Autodesk Fusion 360 part; units mm, degrees
note: some values were not read from the file. Chosen so that the rebuilt part matches the saved one: which bodies a step acts on; which pieces of a blend or face edit are solid. Set by a fixed rule: which sketch regions a step uses.
(part 4 of 4)
  spline S28 degree 5 poles (-8.8975, 18.3699) (-8.9029, 18.3732) (-8.9137, 18.3794) (-8.9303, 18.3884) (-8.9529, 18.3994) (-8.9818, 18.4118) (-9.0111, 18.4234) (-9.0408, 18.4344) (-9.0706, 18.4451) (-9.1006, 18.4555) (-9.1307, 18.4658) (-9.1609, 18.4758) (-9.1914, 18.4854) (-9.222, 18.4945) (-9.2529, 18.5032) (-9.284, 18.5115) (-9.3152, 18.5194) (-9.3466, 18.527) (-9.3782, 18.5343) (-9.4098, 18.5413) (-9.4416, 18.5482) (-9.4735, 18.5547) (-9.5055, 18.5609) (-9.5376, 18.5669) (-9.5699, 18.5726) (-9.6023, 18.578) (-9.6348, 18.5831) (-9.6674, 18.588) (-9.7002, 18.5926) (-9.733, 18.597) (-9.7659, 18.6011) (-9.7989, 18.605) (-9.832, 18.6087) (-9.8652, 18.6121) (-9.8985, 18.6152) (-9.9319, 18.6182) (-9.9654, 18.6209) (-9.9989, 18.6233) (-10.0326, 18.6256) (-10.0663, 18.6276) (-10.1001, 18.6294) (-10.134, 18.631) (-10.1679, 18.6323) (-10.2019, 18.6334) (-10.236, 18.6344) (-10.2702, 18.635) (-10.3044, 18.6355) (-10.3387, 18.6358) (-10.3731, 18.6358) (-10.4075, 18.6357) (-10.442, 18.6353) (-10.4766, 18.6347) (-10.5112, 18.6339) (-10.5459, 18.6329) (-10.5806, 18.6317) (-10.6154, 18.6303) (-10.6503, 18.6287) (-10.6852, 18.6269) (-10.7202, 18.6249) (-10.7552, 18.6227) (-10.7902, 18.6203) (-10.8253, 18.6176) (-10.8605, 18.6148) (-10.8957, 18.6118) (-10.931, 18.6086) (-10.9663, 18.6052) (-11.0016, 18.6016) (-11.037, 18.5978) (-11.0724, 18.5938) (-11.1079, 18.5896) (-11.1434, 18.5852) (-11.1718, 18.5816) (-11.1932, 18.5787) (-11.2074, 18.5768) (-11.2145, 18.5758) knots 0 0 0 0 0 0 0.01428571 0.02857143 0.04285714 0.05714286 0.07142857 0.08571429 0.1 0.11428571 0.12857143 0.14285714 0.15714286 0.17142857 0.18571429 0.2 0.21428571 0.22857143 0.24285714 0.25714286 0.27142857 0.28571429 0.3 0.31428571 0.32857143 0.34285714 0.35714286 0.37142857 0.38571429 0.4 0.41428571 0.42857143 0.44285714 0.45714286 0.47142857 0.48571429 0.5 0.51428571 0.52857143 0.54285714 0.55714286 0.57142857 0.58571429 0.6 0.61428571 0.62857143 0.64285714 0.65714286 0.67142857 0.68571429 0.7 0.71428571 0.72857143 0.74285714 0.75714286 0.77142857 0.78571429 0.8 0.81428571 0.82857143 0.84285714 0.85714286 0.87142857 0.88571429 0.9 0.91428571 0.92857143 0.94285714 0.95714286 0.97142857 0.98571429 1 1 1 1 1 1
  arc A58 (-11.2145, 18.5758) -> (-11.6071, 17.6942) centre (0, 13.0546) ccw
  spline S29 degree 5 poles (-11.6071, 17.6942) (-11.603, 17.6883) (-11.5949, 17.6764) (-11.5827, 17.6586) (-11.5664, 17.6351) (-11.5459, 17.6057) (-11.5253, 17.5766) (-11.5046, 17.5476) (-11.4837, 17.5187) (-11.4628, 17.4901) (-11.4417, 17.4616) (-11.4205, 17.4332) (-11.3991, 17.405) (-11.3777, 17.377) (-11.3562, 17.3492) (-11.3345, 17.3215) (-11.3127, 17.294) (-11.2908, 17.2667) (-11.2688, 17.2395) (-11.2467, 17.2125) (-11.2244, 17.1857) (-11.2021, 17.1591) (-11.1796, 17.1327) (-11.157, 17.1064) (-11.1344, 17.0803) (-11.1115, 17.0545) (-11.0886, 17.0288) (-11.0656, 17.0032) (-11.0424, 16.9779) (-11.0192, 16.9528) (-10.9958, 16.9279) (-10.9723, 16.9031) (-10.9487, 16.8786) (-10.925, 16.8543) (-10.9011, 16.8302) (-10.8772, 16.8063) (-10.8531, 16.7825) (-10.829, 16.759) (-10.8047, 16.7358) (-10.7803, 16.7127) (-10.7558, 16.6898) (-10.7311, 16.6672) (-10.7064, 16.6448) (-10.6815, 16.6227) (-10.6565, 16.6007) (-10.6314, 16.5791) (-10.6062, 16.5576) (-10.5809, 16.5364) (-10.5554, 16.5154) (-10.5299, 16.4947) (-10.5042, 16.4742) (-10.4784, 16.454) (-10.4524, 16.4341) (-10.4264, 16.4145) (-10.4002, 16.3952) (-10.3738, 16.3761) (-10.3474, 16.3573) (-10.3209, 16.3388) (-10.2942, 16.3205) (-10.2674, 16.3026) (-10.2405, 16.285) (-10.2134, 16.2679) (-10.1861, 16.2512) (-10.1586, 16.235) (-10.1309, 16.2192) (-10.1032, 16.2037) (-10.0753, 16.1885) (-10.0474, 16.1735) (-10.0194, 16.1588) (-9.9912, 16.1447) (-9.9626, 16.1316) (-9.9393, 16.1221) (-9.9216, 16.1158) (-9.9096, 16.1119) (-9.9036, 16.1101) knots -1 -1 -1 -1 -1 -1 -0.98571429 -0.97142857 -0.95714286 -0.94285714 -0.92857143 -0.91428571 -0.9 -0.88571429 -0.87142857 -0.85714286 -0.84285714 -0.82857143 -0.81428571 -0.8 -0.78571429 -0.77142857 -0.75714286 -0.74285714 -0.72857143 -0.71428571 -0.7 -0.68571429 -0.67142857 -0.65714286 -0.64285714 -0.62857143 -0.61428571 -0.6 -0.58571429 -0.57142857 -0.55714286 -0.54285714 -0.52857143 -0.51428571 -0.5 -0.48571429 -0.47142857 -0.45714286 -0.44285714 -0.42857143 -0.41428571 -0.4 -0.38571429 -0.37142857 -0.35714286 -0.34285714 -0.32857143 -0.31428571 -0.3 -0.28571429 -0.27142857 -0.25714286 -0.24285714 -0.22857143 -0.21428571 -0.2 -0.18571429 -0.17142857 -0.15714286 -0.14285714 -0.12857143 -0.11428571 -0.1 -0.08571429 -0.07142857 -0.05714286 -0.04285714 -0.02857143 -0.01428571 0 0 0 0 0 0
  line L29 (-9.9036, 16.1101) -> (-9.6476, 16.0311)
  arc A59 (-9.1027, 15.0919) -> (-9.6476, 16.0311) centre (-9.8834, 15.2666) ccw
  circle A60 centre (0, 13.0546) radius 2
  line L30 (-1.664, 11.945) -> (1.836, 11.945)
  dimension "d55" = 4
  dimension "d56" = 3.5
  constraint concentric A0 A60
  constraint coincident A60 L30.start
  constraint horizontal L30
  measures "d55" diameter of A60
  measures "d56" distance of L30.start L30.end
extrude "Extrude13" cut sketch "Sketch8" against normal blind 4 contours A60 L30 picked at (0.1008, 13.0647) bodies 2
move_body "Move12" bodies 2 to x (1, 0, 0) y (0, 0, -1) z (0, 1, 0) at (0, 0, 0)
move_body "Move13" bodies 2 to x (1, 0, 0) y (0, 1, 0) z (0, 0, 1) at (0, -15, 35)
move_body "Move14" bodies 1 to x (1, 0, 0) y (0, 1, 0) z (0, 0, 1) at (0, -10, -10)
move_body "Move15" bodies 1 to x (1, 0, 0) y (0, 1, 0) z (0, 0, 1) at (0, -7, -2)
named bodies: "Spur Gear (15 teeth)", "Spur Gear (15 teeth) (1)", "Spur Gear (15 teeth) (2)"
